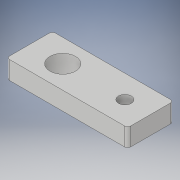
# Autodesk Inventor part: Transmisor_grande
Saved by Autodesk Inventor 2019 (Build 230136000, 136)
## iProperties
Created: 2019-09-30
Part Number: Transmisor_grande
Material: Generic
Document SubType Name: Modeling
Designer: Domenico
Density: 1 g/cm^3
Appearance: Default
Author: Domenico
Autodesk Inventor part; units mm, degrees
ref_plane "YZ Plane" through (0, 0, 0) normal (1, 0, 0) x (0, 1, 0)
ref_plane "XZ Plane" through (0, 0, 0) normal (0, 1, 0) x (-1, 0, 0)
ref_plane "XY Plane" through (0, 0, 0) normal (0, 0, 1) x (1, 0, 0)
sketch "Sketch1" plane through (0, 0, 0) normal (0, 1, 0) x (-1, 0, 0)
  line L0 (0, 0) -> (-120, 0)
  line L1 (-120, 0) -> (-120, -45.4)
  line L2 (-120, -45.4) -> (0, -45.4)
  line L3 (0, -45.4) -> (0, 0)
  circle A0 centre (-33, -22.7) radius 12.7
  circle A1 centre (-94.6, -22.7) radius 6.35
  point P0 (0, -22.7)
  point P1 (-120, -22.7)
  dimension "d0" = 120
  dimension "d1" = 45.4
  dimension "d2" = 33
  dimension "d3" = 25.4
  dimension "d4" = 25.4
  dimension "Diametro_eje_pequeño" = 12.7
  constraints: 8 end point, 2 centre point, 2 horizontal alignment, 2 midpoint, 2 parallel, 1 horizontal, 1 perpendicular
  measures "d0" distance of L2.end L1.end
  measures "d1" distance of L0.end L1.end
  measures "d2" distance from line of L3 A0.centre
  measures "d3" diameter of A0
  measures "d4" distance from line of L1 A1.centre
  measures "Diametro_eje_pequeño" diameter of A1
extrude "Extrusion1" add sketch "Sketch1" along normal blind 18
fillet "Fillet1" radius 3 4 edges at (0, 9, 0) (120, 9, 0) (120, 9, -45.4) (0, 9, -45.4)
equation "\"d1\" = ancho"
equation "\"d2\" = separacion_grande"
equation "\"d3\" = diametro_externo"
equation "\"d4\" = d3"
equation "\"Diametro_eje_pequeño\" = Diametro_eje_pequeño_1"
equation "\"ancho\" = 45.4"
equation "\"separacion_grande\" = 33"
equation "\"diametro_externo\" = 25.4"
equation "\"Diametro_eje_pequeño_1\" = 12.7"
body "Solid1"
